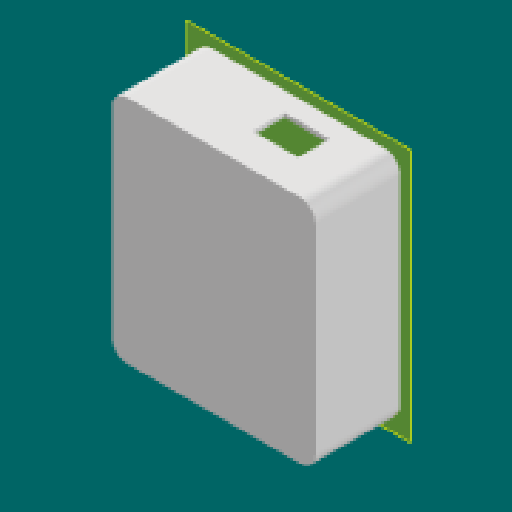
# Autodesk Inventor part: Part2
Saved by Autodesk Inventor 2025.2 (Build 292293000, 293)
## iProperties
Created: 2025-05-30
Part Number: Part2
Material: Generic
Document SubType Name: Modeling
Designer: ia088
Density: 1 g/cm^3
Appearance: Default
Author: ia088
Autodesk Inventor part; units mm, degrees
ref_plane "YZ Plane" through (0, 0, 0) normal (1, 0, 0) x (0, 1, 0)
ref_plane "XZ Plane" through (0, 0, 0) normal (0, 1, 0) x (-1, 0, 0)
ref_plane "XY Plane" through (0, 0, 0) normal (0, 0, 1) x (1, 0, 0)
ref_plane "Work Plane1" through (0, 0, 0) normal (0, 0, 1) x (1, 0, 0)
sketch "Sketch1" plane through (0, 0, 0) normal (0, 0, 1) x (1, 0, 0)
  line L0 (30.375, 39.1) -> (-30.4, 39.1) projected
  arc A0 (34.375, 35.1014) -> (30.375, 39.1) centre (30.375, 35.1) ccw projected
  line L1 (34.4, -35.0986) -> (34.375, 35.1014) projected
  arc A1 (30.4, -39.1) -> (34.4, -35.0986) centre (30.4, -35.1) ccw projected
  line L2 (-30.375, -39.1) -> (30.4, -39.1) projected
  arc A2 (-34.375, -35.1014) -> (-30.375, -39.1) centre (-30.375, -35.1) ccw projected
  line L3 (-34.4, 35.0986) -> (-34.375, -35.1014) projected
  arc A3 (-30.4, 39.1) -> (-34.4, 35.0986) centre (-30.4, 35.1) ccw projected
  arc A4 (-35.875, -35.102) -> (-30.375, -40.6) centre (-30.375, -35.1) ccw projected
  line L4 (30.4, -40.6) -> (-30.375, -40.6) projected
  arc A5 (30.4, -40.6) -> (35.9, -35.098) centre (30.4, -35.1) ccw projected
  line L5 (35.875, 35.102) -> (35.9, -35.098) projected
  arc A6 (35.875, 35.102) -> (30.375, 40.6) centre (30.375, 35.1) ccw projected
  line L6 (-30.4, 40.6) -> (30.375, 40.6) projected
  arc A7 (-30.4, 40.6) -> (-35.9, 35.098) centre (-30.4, 35.1) ccw projected
  line L7 (-35.875, -35.102) -> (-35.9, 35.098) projected
  point P0 (0, 0)
extrude "Extrusion1" add sketch "Sketch1" along normal blind 27.93
sketch "Sketch2" plane through (0, 0, 27.93) normal (0, 0, 1) x (1, 0, 0)
  line L0 (-35.9, 35.098) -> (-35.875, -35.102) projected
  arc A0 (-35.875, -35.102) -> (-30.375, -40.6) centre (-30.375, -35.1) ccw projected
  line L1 (-30.375, -40.6) -> (30.4, -40.6) projected
  arc A1 (30.4, -40.6) -> (35.9, -35.098) centre (30.4, -35.1) ccw projected
  line L2 (35.9, -35.098) -> (35.875, 35.102) projected
  arc A2 (35.875, 35.102) -> (30.375, 40.6) centre (30.375, 35.1) ccw projected
  line L3 (30.375, 40.6) -> (-30.4, 40.6) projected
  arc A3 (-30.4, 40.6) -> (-35.9, 35.098) centre (-30.4, 35.1) ccw projected
  point P0 (0, 0)
extrude "Extrusion2" add sketch "Sketch2" along normal blind 2
sketch "Sketch3" plane through (-30.4, 40.6, 0) normal (0, 1, 0) x (1, 0, 0)
  line L0 (48.3031, -6.91) -> (17.8231, -6.91) projected
  line L1 (48.3031, -6.91) -> (48.3031, -18.01) projected
  line L2 (17.8231, -6.91) -> (17.8231, -18.01) projected
  line L3 (48.3031, -18.01) -> (17.8231, -18.01)
  line L4 (48.3031, -18.01) -> (32.3031, -18.01)
  line L5 (32.3031, -18.01) -> (32.3031, -6.91)
  point P0 (30.4, 0)
  dimension "d9" = 16
  constraints: 6 end point, 2 point on line, 1 horizontal, 1 perpendicular
  measures "d9" distance of L1.end L4.end
extrude "Extrusion3" cut sketch "Sketch3" against normal blind 7.45 contours L1 L3 L5 L0
sketch "Sketch4" plane through (-30.375, -40.6, 0) normal (0, -1, 0) x (1, 0, 0)
  line L0 (17.0619, 6.91) -> (17.0619, 18.01) projected
  line L1 (32.3019, 6.91) -> (17.0619, 6.91) projected
  line L2 (49.2019, 6.91) -> (33.9619, 6.91) projected
  line L3 (49.2019, 6.91) -> (49.2019, 18.01) projected
  line L4 (17.0619, 18.01) -> (49.2019, 18.01)
  line L5 (32.3019, 6.91) -> (33.9619, 6.91)
  line L6 (-0.025, 0) -> (60.75, 0) projected
  line L7 (49.4019, 18.21) -> (49.4019, 6.71)
  line L8 (49.4019, 6.71) -> (33.9619, 6.71)
  line L9 (33.9619, 6.71) -> (32.3019, 6.71)
  line L10 (32.3019, 6.71) -> (16.8619, 6.71)
  line L11 (16.8619, 6.71) -> (16.8619, 18.21)
  line L12 (16.8619, 18.21) -> (49.4019, 18.21)
  point P0 (30.375, 0)
  dimension "d6" = 0.2
  constraints: 16 end point, 1 horizontal, 1 parallel, 5 other
  measures "d6" distance between parallel lines of L4 L12
extrude "Extrusion4" cut sketch "Sketch4" against normal blind 7.45 contours L0 L4 L3 L2 L5 L1 | L7 L8 L9 L10 L11 L12
body "Solid1"
